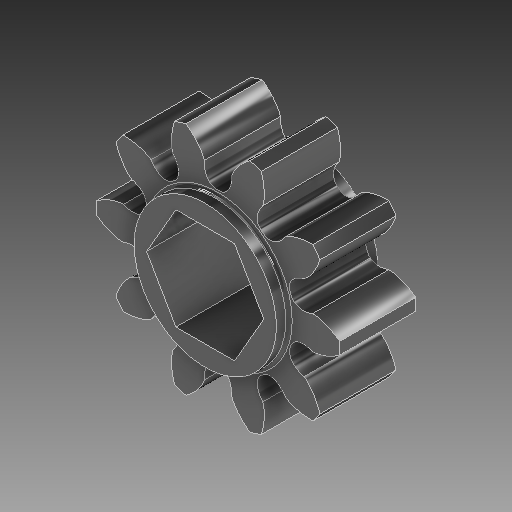
# Autodesk Inventor part: VexPro 10T 10DP 20degPA Gear
Saved by Autodesk Inventor 2022 (Build 260153000, 153)
## iProperties
Created: 2021-10-01
Part Number: VexPro 10T 10DP 20degPA Gear
Material: Steel
Document SubType Name: Modeling
Designer: Max Boord
Density: 7.85 g/cm^3
Appearance: Glazed - Black
Mass: 28.6381 g
Surface Area: 28.8999 cm^2
Volume: 3.64816 cm^3
Author: Max Boord
Autodesk Inventor part; units mm, degrees
ref_plane "YZ Plane" through (0, 0, 0) normal (1, 0, 0) x (0, 1, 0)
ref_plane "XZ Plane" through (0, 0, 0) normal (0, 1, 0) x (-1, 0, 0)
ref_plane "XY Plane" through (0, 0, 0) normal (0, 0, 1) x (1, 0, 0)
sketch "Sketch1" plane through (0, 0, 0) normal (0, 0, 1) x (1, 0, 0)
  spline S0 degree 3 poles (-3.994, 14.7073) (-3.8713, 14.6146) (-3.6258, 14.4291) (-3.2768, 14.1268) (-2.944, 13.8068) (-2.6318, 13.4667) (-2.3432, 13.1062) (-2.1267, 12.7879) (-1.9719, 12.5219) (-1.8672, 12.3163) (-1.7736, 12.105) (-1.7288, 11.9578) (-1.7064, 11.8842) knots 0 0 0 0 0.125009 0.250018 0.375026 0.500029 0.625027 0.750014 0.81252 0.875024 0.937523 1 1 1 1
  spline S1 degree 3 poles (-1.7064, 11.8842) (-1.7089, 11.8148) (-1.7138, 11.6761) (-1.7086, 11.4679) (-1.692, 11.2603) (-1.6589, 11.0547) (-1.6184, 10.8504) (-1.5563, 10.6514) (-1.4808, 10.4573) (-1.386, 10.2715) (-1.2707, 10.0977) (-1.1361, 9.9385) (-0.9811, 9.7986) (-0.8065, 9.6843) (-0.6174, 9.5957) (-0.4493, 9.5507) (-0.3123, 9.5279) (-0.1734, 9.5229) (0, 9.5264) (0.1734, 9.5229) (0.3123, 9.5279) (0.4493, 9.5507) (0.6174, 9.5957) (0.8065, 9.6843) (0.9811, 9.7986) (1.1361, 9.9385) (1.2707, 10.0977) (1.386, 10.2715) (1.4808, 10.4573) (1.5563, 10.6514) (1.6184, 10.8504) (1.6589, 11.0547) (1.692, 11.2603) (1.7086, 11.4679) (1.7138, 11.6761) (1.7089, 11.8148) (1.7064, 11.8842) knots 0 0 0 0 0.020814 0.041627 0.06244 0.083251 0.104061 0.124873 0.14568 0.166493 0.187304 0.208108 0.228908 0.249703 0.270497 0.291281 0.301692 0.312096 0.33291 0.353723 0.364128 0.374538 0.395323 0.416117 0.436912 0.457712 0.478516 0.499327 0.52014 0.540947 0.561759 0.582569 0.60338 0.624193 0.645006 0.66582 0.66582 0.66582 0.66582
  spline S2 degree 3 poles (1.7064, 11.8842) (1.7288, 11.9578) (1.7736, 12.105) (1.8672, 12.3163) (1.9719, 12.5219) (2.1267, 12.7879) (2.3432, 13.1062) (2.6318, 13.4667) (2.944, 13.8068) (3.2768, 14.1268) (3.6258, 14.4291) (3.8713, 14.6146) (3.994, 14.7073) knots 0 0 0 0 0.062477 0.124976 0.18748 0.249986 0.374973 0.499971 0.624974 0.749982 0.874991 1 1 1 1
  circle A0 centre (0, 0) radius 9.525 construction
  circle A1 centre (0, 0) radius 11.9341 construction
  circle A2 centre (0, 0) radius 12.7 construction
  circle A3 centre (0, 0) radius 15.24
  point P0 (-3.629, 14.4251)
  point P1 (-3.2795, 14.1239)
  point P2 (-2.9474, 13.8035)
  point P3 (-2.6357, 13.4633)
  point P4 (-2.348, 13.1026)
  point P5 (-2.0896, 12.7205)
  point P6 (-1.9738, 12.5209)
  point P7 (-1.8691, 12.3153)
  point P8 (-1.778, 12.1034)
  point P9 (-1.7117, 11.6761)
  point P10 (-1.7067, 11.468)
  point P11 (-1.6892, 11.2606)
  point P12 (-1.6577, 11.0549)
  point P13 (-1.6148, 10.8513)
  point P14 (-1.5541, 10.6522)
  point P15 (-1.4776, 10.4587)
  point P16 (-1.3826, 10.2735)
  point P17 (-1.2675, 10.1001)
  point P18 (-1.1327, 9.9417)
  point P19 (-0.9778, 9.8028)
  point P20 (-0.8041, 9.6886)
  point P21 (-0.6153, 9.6015)
  point P22 (-0.4149, 9.5461)
  point P23 (-0.312, 9.5302)
  point P24 (-0.2081, 9.5248)
  point P25 (0, 9.525)
  point P26 (0.2081, 9.5248)
  point P27 (0.312, 9.5302)
  point P28 (0.4149, 9.5461)
  point P29 (0.6153, 9.6015)
  point P30 (0.8041, 9.6886)
  point P31 (0.9778, 9.8028)
  point P32 (1.1327, 9.9417)
  point P33 (1.2675, 10.1001)
  point P34 (1.3826, 10.2735)
  point P35 (1.4776, 10.4587)
  point P36 (1.5541, 10.6522)
  point P37 (1.6148, 10.8513)
  point P38 (1.6577, 11.0549)
  point P39 (1.6892, 11.2606)
  point P40 (1.7067, 11.468)
  point P41 (1.7117, 11.6761)
  point P42 (1.778, 12.1034)
  point P43 (1.8691, 12.3153)
  point P44 (1.9738, 12.5209)
  point P45 (2.0896, 12.7205)
  point P46 (2.348, 13.1026)
  point P47 (2.6357, 13.4633)
  point P48 (2.9474, 13.8035)
  point P49 (3.2795, 14.1239)
  point P50 (3.629, 14.4251)
  constraints: 4 centre point, 2 point on circle, 117 other
extrude "Extrusion1" add sketch "Sketch1" along normal mid plane 9.525
extrude "Extrusion2" cut sketch "Sketch1" along normal mid plane 25.4 contours A3 S2 S1 S0 picked at (0.466, 13.3949)
pattern_circular "Circular Pattern1" count 10 over 360 about axis through (0, 0, 0) along (0, 0, 1) of "Extrusion2"
sketch "Sketch2" plane through (0, 0, 4.7625) normal (0, 0, 1) x (1, 0, 0)
  line L0 (-7.3323, 0) -> (-3.6662, 6.35)
  line L1 (-3.6662, 6.35) -> (3.6662, 6.35)
  line L2 (3.6662, 6.35) -> (7.3323, 0)
  line L3 (7.3323, 0) -> (3.6662, -6.35)
  line L4 (3.6662, -6.35) -> (-3.6662, -6.35)
  line L5 (-3.6662, -6.35) -> (-7.3323, 0)
  circle A0 centre (0, 0) radius 8.89
  dimension "d7" = 12.7
  dimension "d8" = 17.78
  constraints: 12 end point, 2 coincident, 1 centre point, 1 horizontal, 13 other
  measures "d7" distance between parallel lines of L4 L1
  measures "d8" diameter of A0
extrude "Extrusion3" cut sketch "Sketch2" against normal blind 25.4 contours L0 L1 L2 L3 L4 L5
extrude "Extrusion4" add sketch "Sketch2" along normal mid plane 12.7 from surface at -4.7625
fillet "Fillet1" radius 0.3969 2 edges at (-8.89, 0, 4.7625) (-8.89, 0, -4.7625)
equation "\"Module\" = 2.54"
equation "\"PressureAngle\" = 20deg"
equation "\"UnitProfileClearance\" = 0.25"
equation "\"UnitRoundRadius\" = 0.35"
equation "\"HeadDiameter\" = 30.48"
equation "\"RootDiameter\" = 19.05"
equation "\"BaseDiameter\" = 23.86819"
equation "\"PitchDiameter\" = 25.4"
equation "\"FaceWidth\" = 3.175"
equation "\"HelixAngle\" = 0"
equation "\"UnitCorrection\" = 0"
equation "\"UnitAddendumModification\" = 0"
equation "\"CircularPitch\" = 7.97965"
equation "\"UnitBacklashShift\" = 0"
equation "\"TotalToolShift\" = 0"
equation "\"IsInternal\" = 0"
body "Solid1"
